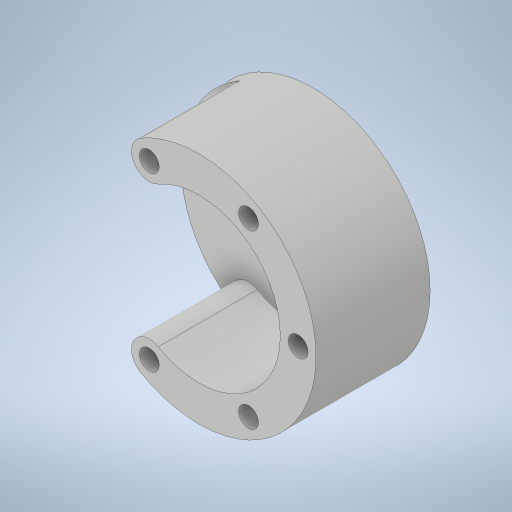
# Autodesk Inventor part: Motor_spacer_Falcon
Saved by Autodesk Inventor 2023.4 (Build 274418000, 418)
## iProperties
Created: 2024-01-19
Part Number: Motor_spacer_Falcon
Material: Generic
Document SubType Name: Modeling
Designer: jmcintyr
Density: 1 g/cm^3
Appearance: Default
Author: jmcintyr
Autodesk Inventor part; units mm, degrees
ref_plane "YZ Plane" through (0, 0, 0) normal (1, 0, 0) x (0, 1, 0)
ref_plane "XZ Plane" through (0, 0, 0) normal (0, 1, 0) x (-1, 0, 0)
ref_plane "XY Plane" through (0, 0, 0) normal (0, 0, 1) x (1, 0, 0)
sketch "Sketch1" plane through (0, 0, 0) normal (0, 0, 1) x (1, 0, 0)
  circle A0 centre (0, 0) radius 29.972
  circle A1 centre (0, 0) radius 25.4 construction
  circle A2 centre (12.7, 21.997) radius 2.5527 construction
  circle A3 centre (-12.7, 21.997) radius 2.5527 construction
  circle A4 centre (-25.4, 0) radius 2.5527 construction
  circle A5 centre (-12.7, -21.997) radius 2.5527 construction
  circle A6 centre (12.7, -21.997) radius 2.5527 construction
  circle A7 centre (25.4, 0) radius 2.5527 construction
  line L0 (-12.7, 21.997) -> (12.7, 21.997) construction
  arc A8 (-14.986, 25.9565) -> (-10.414, 18.0376) centre (-12.7, 21.997) ccw
  arc A9 (-10.414, -18.0376) -> (-10.414, 18.0376) centre (0, 0) ccw
  arc A10 (-10.414, -18.0376) -> (-14.986, -25.9565) centre (-12.7, -21.997) ccw
  dimension "d1" = 50.8
  dimension "d0" = 59.944
  dimension "d2" = 5.1054
  dimension "d5" = 360
  constraints: 10 centre point, 10 point on circle, 5 coincident, 2 end point, 2 tangent, 1 equal radius, 1 horizontal, 16 other
  measures "d0" diameter of A0
  measures "d2" diameter of A2
extrude "Extrusion1" add sketch "Sketch1" along normal blind 25.4 contours A0 A10 A9 A8 picked at (-11.332, -24.2357)
sketch "Sketch2" plane through (0, 0, 0) normal (0, 0, -1) x (-1, 0, 0)
  circle A0 centre (0, 0) radius 29.972
  circle A1 centre (0, 0) radius 9.8425
  arc A2 (14.986, 25.9565) -> (14.986, -25.9565) centre (0, 0) ccw projected
  dimension "d13" = 19.685
  dimension "d14" = 59.944
  constraints: 2 centre point, 2 coincident
  measures "d13" diameter of A1
  measures "d14" diameter of A0
extrude "Extrusion2" add sketch "Sketch2" along normal blind 3.81
sketch "Sketch3" plane through (0, 0, 25.4) normal (0, 0, 1) x (1, 0, 0)
  circle A0 centre (0, 0) radius 9.8425 projected
  circle A1 centre (0, 0) radius 25.4
  arc A2 (-14.986, 25.9565) -> (-10.414, 18.0376) centre (-12.7, 21.997) ccw projected
  point P0 (-25.4, 0)
  point P1 (-12.7, -21.997)
  point P2 (12.7, -21.997)
  point P3 (25.4, 0)
  point P4 (12.7, 21.997)
  dimension "d19" = 360
  constraints: 2 coincident, 10 other
hole "Hole1" at (-12.7, 21.997, 25.4) at (12.7, 21.997, 25.4) at (25.4, 0, 25.4) at (12.7, -21.997, 25.4) at (-12.7, -21.997, 25.4) direction (0, 0, -1) diameter 5.1054 end through all
body "Solid1"
